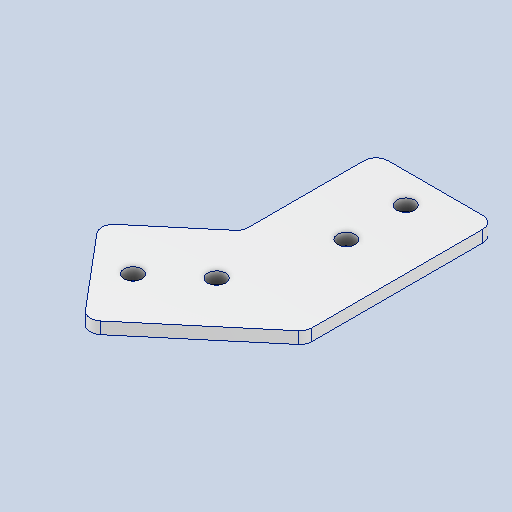
# Autodesk Inventor part: base_weel-v3-Plate-10
Saved by Autodesk Inventor 2025.2 (Build 292293000, 293)
## iProperties
Created: 2025-04-05
Part Number: base_weel-v3-Plate-10
Material: アルミニウム 6061
Document SubType Name: Modeling
Designer: haruy
Density: 2.7 g/cm^3
Appearance: アルミニウム - フラット
Author: haruy
Autodesk Inventor part; units mm, degrees
ref_plane "YZ Plane" through (0, 0, 0) normal (1, 0, 0) x (0, 1, 0)
ref_plane "XZ Plane" through (0, 0, 0) normal (0, 1, 0) x (-1, 0, 0)
ref_plane "XY Plane" through (0, 0, 0) normal (0, 0, 1) x (1, 0, 0)
derived "base_weel-v3-ASP-Base.ipt"
sketch "スケッチ8" plane through (0, -300, -190) normal (0, -1, 0) x (1, 0, 0)
  line L0 (47.5, 215) -> (12.5, 215) projected
  line L1 (12.5, 215) -> (12.5, 165) projected
  line L2 (12.5, 165) -> (47.5, 165) projected
  line L3 (47.5, 165) -> (47.5, 215) projected
  line L4 (12.5, 212) -> (-22.5, 212) projected
  line L5 (-22.5, 212) -> (-22.5, 168) projected
  line L6 (-22.5, 168) -> (12.5, 168) projected
  line L7 (12.5, 168) -> (12.5, 212) projected
  line L8 (-32.5, 456.6712) -> (-32.5, -73.3765) projected
  line L9 (-20, 0) -> (-20, 380) projected
  line L10 (-16.5, 212) -> (-16.5, 168) projected
  line L11 (0, 238.5) -> (20, 238.5) projected
  line L12 (0, 141.5) -> (20, 141.5) projected
  line L13 (47.5, 220) -> (52.5, 220) projected
  line L14 (52.5, 220) -> (52.5, 160) projected
  line L15 (52.5, 160) -> (47.5, 160) projected
  line L16 (47.5, 160) -> (47.5, 220) projected
  line L17 (52.5, 245) -> (72.5, 245) projected
  line L18 (72.5, 245) -> (72.5, 135) projected
  line L19 (72.5, 135) -> (52.5, 135) projected
  line L20 (52.5, 135) -> (52.5, 245) projected
  line L21 (-20, 288.5) -> (0, 288.5) projected
  line L22 (0, 288.5) -> (0, 268.5) projected
  line L23 (0, 268.5) -> (-20, 268.5) projected
  line L24 (-20, 268.5) -> (-20, 288.5) projected
  line L25 (-20, 91.5) -> (0, 91.5) projected
  line L26 (0, 91.5) -> (0, 111.5) projected
  line L27 (0, 111.5) -> (-20, 111.5) projected
  line L28 (-20, 111.5) -> (-20, 91.5) projected
  line L29 (52.5, 220) -> (-27.5375, 220) projected
  line L30 (-27.5375, 220) -> (-27.5375, 225) projected
  line L31 (-27.5375, 225) -> (52.5, 225) projected
  line L32 (52.5, 225) -> (52.5, 220) projected
  line L33 (1.0432, 290.7771) -> (54.5886, 245.6896) projected
  line L34 (54.5886, 245.6896) -> (67.4708, 260.9882) projected
  line L35 (67.4708, 260.9882) -> (13.9254, 306.0758) projected
  line L36 (13.9254, 306.0758) -> (1.0432, 290.7771) projected
  line L37 (-22.5, 190) -> (47.5, 190) projected
  line L38 (52.1721, 273.8704) -> (39.2899, 258.5717) projected
  line L39 (29.2241, 293.1937) -> (16.3419, 277.895) projected
  line L40 (1.0432, 89.2229) -> (54.5886, 134.3104) projected
  line L41 (13.9254, 73.9242) -> (1.0432, 89.2229) projected
  line L42 (54.5886, 134.3104) -> (67.4708, 119.0118) projected
  line L43 (67.4708, 119.0118) -> (13.9254, 73.9242) projected
  line L44 (52.5, 245) -> (52.5, 135) projected
  line L45 (52.5, 135) -> (72.5, 135) projected
  line L46 (72.5, 135) -> (72.5, 245) projected
  line L47 (72.5, 245) -> (52.5, 245) projected
  line L48 (0, 380) -> (0, 0) projected
  line L49 (0, 263.5) -> (-20, 263.5) projected
  line L50 (0, 116.5) -> (-20, 116.5) projected
  line L51 (-20, 263.5) -> (0, 263.5) projected
  line L52 (0, 263.5) -> (0, 116.5) projected
  line L53 (0, 116.5) -> (-20, 116.5) projected
  line L54 (-20, 116.5) -> (-20, 263.5) projected
  line L55 (0, 288.5) -> (3.7475, 288.5) projected
  line L56 (0, 317.8016) -> (-20, 317.8016) projected
  circle A0 centre (-10, 298.5) radius 1.5 projected
  circle A1 centre (-10, 308.5) radius 1.5 projected
  line L57 (13.9254, 306.0758) -> (0, 317.8016) projected
  circle A2 centre (11.309, 295.2059) radius 1.5 projected
  circle A3 centre (18.9583, 288.7648) radius 1.5 projected
  line L58 (52.5, 245) -> (52.5, 247.4483) projected
  line L59 (67.4708, 260.9882) -> (83.3351, 247.6298) projected
  line L60 (72.5, 245) -> (72.5, 262.2723) projected
  line L61 (72.5, 225) -> (52.5, 225) projected
  circle A4 centre (49.5557, 263.0005) radius 1.5 projected
  circle A5 centre (57.205, 256.5594) radius 1.5 projected
  circle A6 centre (62.5, 240) radius 1.5 projected
  circle A7 centre (62.5, 230) radius 1.5 projected
  circle A8 centre (62.5, 140) radius 1.5 projected
  circle A9 centre (62.5, 150) radius 1.5 projected
  circle A10 centre (57.205, 123.4406) radius 1.5 projected
  circle A11 centre (49.5557, 116.9995) radius 1.5 projected
  circle A12 centre (-10, 71.5) radius 1.5 projected
  circle A13 centre (-10, 81.5) radius 1.5 projected
  circle A14 centre (11.309, 84.7941) radius 1.5 projected
  circle A15 centre (18.9583, 91.2352) radius 1.5 projected
  point P0 (0, 190)
  point P1 (72.5, 256.7534)
  constraints: 1 other
extrude "押し出し1" add sketch "スケッチ8" along normal blind 2 contours L20 L17 L18 L61 | L58 L33 L34 L59 L60 L17 | L33 L38 L35 L34
fillet "フィレット1" radius 2 6 edges at (52.1721, -301, 83.8704) (72.5, -301, 66.7534) (72.5, -301, 35) (39.2899, -301, 68.5717) (52.5, -301, 57.4483) (52.5, -301, 35)
